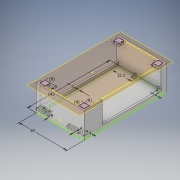
# Autodesk Inventor part: rumba_frame_mount
Saved by Autodesk Inventor 2019.1 (Build 231200000, 200)
## iProperties
Created: 2018-07-25
Part Number: rumba_frame_mount
Material: Generic
Document SubType Name: Modeling
Designer: verdammte
Density: 1 g/cm^3
Appearance: Default
Author: verdammte
Autodesk Inventor part; units mm, degrees
ref_plane "YZ Plane" through (0, 0, 0) normal (1, 0, 0) x (0, 1, 0)
ref_plane "XZ Plane" through (0, 0, 0) normal (0, 1, 0) x (-1, 0, 0)
ref_plane "XY Plane" through (0, 0, 0) normal (0, 0, 1) x (1, 0, 0)
sketch "Sketch1" plane through (0, 0, 0) normal (0, 1, 0) x (-1, 0, 0)
  line L0 (32.5791, 64.9096) -> (-50.4209, 64.9096)
  line L1 (-50.4209, 64.9096) -> (-50.4209, -78.0904)
  line L2 (-50.4209, -78.0904) -> (32.5791, -78.0904)
  line L3 (32.5791, -78.0904) -> (32.5791, 64.9096)
  line L4 (29.5791, 61.9096) -> (-47.4209, 61.9096)
  line L5 (-47.4209, 61.9096) -> (-47.4209, -75.0904)
  line L6 (-47.4209, -75.0904) -> (29.5791, -75.0904)
  line L7 (29.5791, -75.0904) -> (29.5791, 61.9096)
  line L8 (29.5791, -75.0904) -> (29.5791, -78.0904)
  line L9 (-47.4209, -70.2006) -> (-50.4209, -70.2006)
  line L10 (-47.4209, 33.4969) -> (-50.4209, 33.4969)
  line L11 (29.5791, 57.9608) -> (32.5791, 57.9608)
  line L12 (29.5791, -75.0904) -> (32.5791, -75.0904)
  point P0 (0, 0)
  dimension "d0" = 143
  dimension "d1" = 83
  dimension "d2" = 3
  constraints: 26 end point, 9 point on line, 6 perpendicular, 4 parallel, 1 horizontal, 3 other
  measures "d0" distance of L2.end L0.start
  measures "d1" distance of L0.start L0.end
  measures "d2" distance between parallel lines of L3 L7
extrude "Floor" add sketch "Sketch1" along normal blind 3
extrude "Walls" add sketch "Sketch1" along normal blind 20 contours L3 L11 L7 L4 L5 L10 L1 L0 | L3 L12 L7 L11 | L10 L5 L9 L1 | L3 L2 L8 L12 | L9 L5 L6 L8 L2 L1
sketch "Sketch2" plane through (0, 0, 0) normal (0, 1, 0) x (-1, 0, 0)
  line L0 (-47.4209, 61.9096) -> (29.5791, 61.9096) projected
  line L1 (29.5791, -75.0904) -> (-47.4209, -75.0904) projected
  line L2 (29.5791, 61.9096) -> (29.5791, -75.0904) projected
  line L3 (-47.4209, -75.0904) -> (-47.4209, 61.9096) projected
  circle A0 centre (25.5791, 57.9096) radius 2.5
  circle A1 centre (-43.4209, 57.9096) radius 2.5
  circle A2 centre (-43.4209, -71.0904) radius 2.5
  circle A3 centre (-2.5209, -71.0904) radius 2.5
  line L4 (-47.4209, 61.9096) -> (-47.4209, -75.0904) projected
  line L5 (-47.4209, -68.5904) -> (-50.4209, -68.5904)
  line L6 (-50.4209, -68.5904) -> (-50.4209, 27.9367)
  line L7 (-50.4209, 64.9096) -> (-50.4209, -78.0904) projected
  line L8 (-47.4209, 27.9367) -> (-50.4209, 27.9367)
  line L9 (29.5791, -75.0904) -> (29.5791, 61.9096) projected
  line L10 (29.5791, 55.4096) -> (32.4454, 55.4096)
  line L11 (-47.4209, -75.0904) -> (29.5791, -75.0904) projected
  line L12 (29.5791, -75.0904) -> (29.5791, -78.0904)
  point P0 (0, 0)
  dimension "d30" = 4
  dimension "d31" = 4
  dimension "d32" = 4
  dimension "d33" = 4
  dimension "d34" = 4
  dimension "d35" = 4
  dimension "d36" = 4
  dimension "d37" = 32.1
  constraints: 10 end point, 4 centre point, 4 coincident, 4 point on line, 2 horizontal, 1 perpendicular, 1 vertical
  measures "d30" distance from line of L0 A0.centre
  measures "d31" distance from line of L0 A1.centre
  measures "d32" distance from line of L1 A2.centre
  measures "d33" distance from line of L1 A3.centre
  measures "d34" distance from line of L2 A0.centre
  measures "d35" distance from line of L3 A1.centre
  measures "d36" distance from line of L3 A2.centre
  measures "d37" distance from line of L2 A3.centre
extrude "mounts" add sketch "Sketch2" along normal blind 8 contours A0 | A1 | A2 | A3
hole "Hole1" at (43.4209, 0, -71.0904) at (43.4209, 0, 57.9096) at (2.5209, 0, -71.0904) at (-25.5791, 0, 57.9096) direction (0, 1, 0) diameter 3 depth 8
extrude "Extrusion5" cut sketch "Sketch1" along normal blind 20 contours L10 L5 L9 L1
extrude "Extrusion6" cut sketch "Sketch1" along normal blind 20 contours L3 L12 L7 L11 | L3 L2 L8 L12
extrude "Extrusion7" add sketch "Sketch1" along normal blind 8 contours L10 L5 L9 L1
extrude "Extrusion8" add sketch "Sketch1" along normal blind 8 contours L3 L12 L7 L11 | L3 L2 L8 L12
sketch "Sketch3" plane through (-32.5791, 0, 64.9096) normal (0, 0, 1) x (1, 0, 0)
  line L0 (0, 0) -> (0, 20) construction
  line L1 (0, 10) -> (97.9753, 10) construction
  line L2 (0, 20) -> (83, 20) construction
  line L3 (5.9967, 10) -> (23.1011, 10) construction
  line L4 (5.9967, 7.25) -> (23.1011, 7.25)
  line L5 (23.1011, 12.75) -> (5.9967, 12.75)
  arc A0 (5.9967, 12.75) -> (5.9967, 7.25) centre (5.9967, 10) ccw
  arc A1 (23.1011, 7.25) -> (23.1011, 12.75) centre (23.1011, 10) ccw
  line L6 (75.4862, 10) -> (58.3819, 10) construction
  line L7 (75.4862, 12.5) -> (58.3819, 12.5)
  line L8 (58.3819, 7.5) -> (75.4862, 7.5)
  arc A2 (75.4862, 7.5) -> (75.4862, 12.5) centre (75.4862, 10) ccw
  arc A3 (58.3819, 12.5) -> (58.3819, 7.5) centre (58.3819, 10) ccw
  line L9 (0, 0) -> (83, 0) projected
  point P0 (32.5791, 0)
  point P1 (14.5489, 10)
  point P2 (66.9341, 10)
  point P3 (40.0449, 10)
  dimension "d59" = 5.5
  dimension "d60" = 5
  dimension "d80" = 10
  dimension "d81" = 10
  constraints: 18 end point, 8 point on circle, 8 tangent, 5 parallel, 5 point on line, 4 centre point, 3 midpoint
  measures "d59" diameter of A1
  measures "d60" diameter of A3
  measures "d80" distance from line of L9 point (14.549, 10)
  measures "d81" distance from line of L9 point (66.934, 10)
extrude "Extrusion9" add sketch "Sketch3" along normal blind 4.2
chamfer "Chamfer1" distance 1.25 angle 45 8 edges at (-6.7281, 10, 69.1096) (-18.0302, 12.75, 69.1096) (-29.3324, 10, 69.1096) (-18.0302, 7.25, 69.1096) (45.4071, 10, 69.1096) (34.3549, 12.5, 69.1096) (23.3027, 10, 69.1096) (34.3549, 7.5, 69.1096)
hole "Hole2" at (8.9209, 10, 64.9096) direction (0, 0, 1) diameter 4 depth 3
extrude "Extrusion10" add sketch "Sketch1" along normal blind 45 contours L3 L11 L7 L4 L5 L10 L1 L0
extrude "Extrusion11" add sketch "Sketch1" along normal blind 45 contours L9 L5 L6 L8 L2 L1
extrude "Extrusion12" add sketch "Sketch1" along normal blind 45 contours L3 L2 L8 L12
ref_plane "Work Plane1" through (47.4209, 45, -75.0904) normal (0, 1, 0) x (1, 0, 0)
sketch "Sketch4" plane through (0, 45, 0) normal (0, 1, 0) x (1, 0, 0)
  line L0 (47.4209, -61.9096) -> (47.4209, 75.0904) projected
  line L1 (47.4209, -61.9096) -> (38.4209, -61.9096)
  line L2 (38.4209, -61.9096) -> (38.4209, -52.9096)
  line L3 (38.4209, -52.9096) -> (47.4209, -52.9096)
  line L4 (47.4209, -52.9096) -> (47.4209, -61.9096)
  line L5 (47.4209, -61.9096) -> (-29.5791, -61.9096) projected
  line L6 (-29.5791, -61.9096) -> (-20.5791, -61.9096)
  line L7 (-20.5791, -61.9096) -> (-20.5791, -52.9096)
  line L8 (-20.5791, -52.9096) -> (-29.5791, -52.9096)
  line L9 (-29.5791, -52.9096) -> (-29.5791, -61.9096)
  line L10 (47.4209, 75.0904) -> (-29.5791, 75.0904) projected
  line L11 (47.4209, 75.0904) -> (38.4209, 75.0904)
  line L12 (38.4209, 75.0904) -> (38.4209, 66.0904)
  line L13 (38.4209, 66.0904) -> (47.4209, 66.0904)
  line L14 (47.4209, 66.0904) -> (47.4209, 75.0904)
  line L15 (-29.5791, 75.0904) -> (-20.5791, 75.0904)
  line L16 (-20.5791, 75.0904) -> (-20.5791, 66.0904)
  line L17 (-20.5791, 66.0904) -> (-29.5791, 66.0904)
  line L18 (-29.5791, 66.0904) -> (-29.5791, 75.0904)
  line L19 (-32.5791, 75.0904) -> (47.4209, 75.0904) projected
  point P0 (0, 0)
  dimension "d84" = 9
  dimension "d85" = 9
  dimension "d86" = 9
  dimension "d87" = 9
  dimension "d88" = 9
  dimension "d89" = 9
  dimension "d90" = 9
  constraints: 32 end point, 12 parallel, 6 point on line, 4 horizontal, 4 perpendicular
  measures "d84" distance of L16.end L17.end
  measures "d85" distance of L15.end L16.end
  measures "d86" distance of L12.end L13.end
  measures "d87" distance of L7.end L8.end
  measures "d88" distance of L6.end L7.end
  measures "d89" distance of L1.end L2.end
  measures "d90" distance of L2.end L3.end
extrude "Extrusion13" add sketch "Sketch4" against normal blind 5 contours L5 L9 L8 L7
extrude "Extrusion14" add sketch "Sketch4" against normal blind 5 contours L1 L2 L3 L0 | L13 L12 L10 L0 | L16 L17 L18 L10
body "Solid1"
